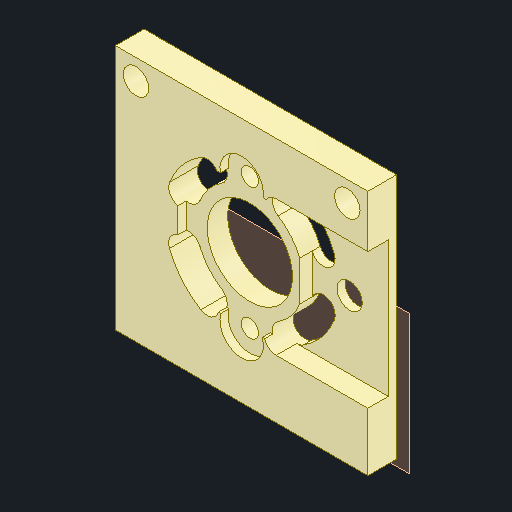
# Autodesk Inventor part: front_motur_holder
Saved by Autodesk Inventor 2023 (Build 270158000, 158)
## iProperties
Created: 2024-04-30
Part Number: front_motur_holder
Material: Nylon 6/6
Document SubType Name: Modeling
Designer: szymo
Density: 1.13 g/cm^3
Appearance: Nylon 6
Mass: 2.38963 g
Surface Area: 22.831 cm^2
Volume: 2.11472 cm^3
Author: szymo
Autodesk Inventor part; units mm, degrees
ref_plane "YZ Plane" through (0, 0, 0) normal (1, 0, 0) x (0, 1, 0)
ref_plane "XZ Plane" through (0, 0, 0) normal (0, 1, 0) x (-1, 0, 0)
ref_plane "XY Plane" through (0, 0, 0) normal (0, 0, 1) x (1, 0, 0)
ref_plane "Work Plane1" through (0, 0, 0) normal (0, 0, 1) x (1, 0, 0)
sketch "Sketch1" plane through (0, 0, 0) normal (0, 0, 1) x (1, 0, 0)
  arc A0 (-3.651, 13.5937) -> (-4.7619, 15.391) centre (-4.2064, 14.4923) ccw projected
  arc A1 (-3.651, 13.5937) -> (-6.4477, 10.2643) centre (0, 7.6875) ccw projected
  arc A2 (-8.4097, 11.0483) -> (-6.4477, 10.2643) centre (-7.4287, 10.6563) ccw projected
  arc A3 (-4.7619, 15.391) -> (-8.4097, 11.0483) centre (0, 7.6875) ccw projected
  arc A4 (6.4477, 10.2643) -> (8.4097, 11.0483) centre (7.4287, 10.6563) ccw projected
  arc A5 (6.4477, 10.2643) -> (3.651, 13.5937) centre (0, 7.6875) ccw projected
  arc A6 (4.7619, 15.391) -> (3.651, 13.5937) centre (4.2064, 14.4923) ccw projected
  arc A7 (8.4097, 11.0483) -> (4.7619, 15.391) centre (0, 7.6875) ccw projected
  arc A8 (-6.4563, 5.1322) -> (-8.4209, 4.3547) centre (-7.4386, 4.7434) ccw projected
  arc A9 (-6.4563, 5.1322) -> (-3.651, 1.7813) centre (0, 7.6875) ccw projected
  arc A10 (-4.7619, -0.016) -> (-3.651, 1.7813) centre (-4.2064, 0.8827) ccw projected
  arc A11 (-8.4209, 4.3547) -> (-4.7619, -0.016) centre (0, 7.6875) ccw projected
  arc A12 (3.651, 1.7813) -> (4.7619, -0.016) centre (4.2064, 0.8827) ccw projected
  arc A13 (3.651, 1.7813) -> (6.4563, 5.1322) centre (0, 7.6875) ccw projected
  arc A14 (8.4209, 4.3547) -> (6.4563, 5.1322) centre (7.4386, 4.7434) ccw projected
  arc A15 (4.7619, -0.016) -> (8.4209, 4.3547) centre (0, 7.6875) ccw projected
  circle A16 centre (10.65, 7.6999) radius 1.15 projected
  circle A17 centre (0, 15.6875) radius 1.0564 projected
  circle A18 centre (0, -0.3125) radius 1.0564 projected
  circle A19 centre (0, 7.6875) radius 5 projected
  circle A20 centre (0, 7.6875) radius 13.7 projected
  line L0 (-116.625, -11.1875) -> (15.375, -11.1875) projected
  line L1 (15.375, -11.1875) -> (15.375, -7.6875) projected
  line L2 (-116.625, -7.6875) -> (15.375, -7.6875) projected
  line L3 (-116.625, -11.1875) -> (-116.625, -7.6875) projected
  line L4 (15.375, -7.6875) -> (-15.375, -7.6875)
  line L5 (-15.375, -7.6875) -> (-15.375, 22.3125)
  line L6 (-15.375, 22.3125) -> (15.375, 22.3125)
  line L7 (15.375, 22.3125) -> (15.375, -7.6875)
  circle A21 centre (0, 7.6875) radius 14.375 projected
  circle A22 centre (0, 7.6875) radius 5.2
  arc A23 (-3.4406, 13.2535) -> (-4.9722, 15.7312) centre (-4.2064, 14.4923) ccw
  arc A24 (-3.4406, 13.2535) -> (-6.0763, 10.1158) centre (0, 7.6875) ccw
  arc A25 (-8.7812, 11.1968) -> (-6.0763, 10.1158) centre (-7.4287, 10.6563) ccw
  arc A26 (-4.9722, 15.7312) -> (-8.7812, 11.1968) centre (0, 7.6875) ccw
  arc A27 (4.9722, 15.7312) -> (3.4406, 13.2535) centre (4.2064, 14.4923) ccw
  arc A28 (6.0763, 10.1158) -> (3.4406, 13.2535) centre (0, 7.6875) ccw
  arc A29 (6.0763, 10.1158) -> (8.7812, 11.1968) centre (7.4287, 10.6563) ccw
  arc A30 (8.7812, 11.1968) -> (4.9722, 15.7312) centre (0, 7.6875) ccw
  arc A31 (3.4406, 2.1215) -> (6.0844, 5.2794) centre (0, 7.6875) ccw
  arc A32 (3.4406, 2.1215) -> (4.9722, -0.3562) centre (4.2064, 0.8827) ccw
  arc A33 (4.9722, -0.3562) -> (8.7928, 4.2075) centre (0, 7.6875) ccw
  arc A34 (8.7928, 4.2075) -> (6.0844, 5.2794) centre (7.4386, 4.7434) ccw
  arc A35 (-6.0844, 5.2794) -> (-8.7928, 4.2075) centre (-7.4386, 4.7434) ccw
  arc A36 (-6.0844, 5.2794) -> (-3.4406, 2.1215) centre (0, 7.6875) ccw
  arc A37 (-4.9722, -0.3562) -> (-3.4406, 2.1215) centre (-4.2064, 0.8827) ccw
  arc A38 (-8.7928, 4.2075) -> (-4.9722, -0.3562) centre (0, 7.6875) ccw
  circle A39 centre (10.65, 7.6999) radius 1.55
  point P0 (0, 0)
  dimension "d0" = 30
  dimension "d1" = 15.375
  dimension "d2" = 15.375
  dimension "d3" = 0.2
  dimension "d4" = 0.4
  dimension "d5" = 0.4
  dimension "d6" = 0.4
  dimension "d7" = 0.4
  dimension "d8" = 0.4
  constraints: 32 point on circle, 18 centre point, 8 end point, 2 parallel, 1 horizontal, 1 perpendicular, 12 other
  measures "d0" distance of L4.end L5.end
  measures "d1" distance from line of A3.centre L7
  measures "d2" distance from line of L5 A1.centre
  measures "d3" radial gap between concentric circles of A19 A22
  measures "d4" radial gap between concentric circles of A0 A23
  measures "d5" radial gap between concentric circles of A7 A30
  measures "d6" radial gap between concentric circles of A14 A34
  measures "d7" radial gap between concentric circles of A8 A35
  measures "d8" radial gap between concentric circles of A16 A39
extrude "Extrusion1" add sketch "Sketch1" along normal blind 1 contours A20 | L2 L5 L6 L7 | A21
sketch "Sketch2" plane through (0, 0, 1) normal (0, 0, 1) x (1, 0, 0)
  line L0 (15.375, 22.3125) -> (-15.375, 22.3125) projected
  line L1 (-15.375, 22.3125) -> (-15.375, -7.6875) projected
  line L2 (-15.375, -7.6875) -> (15.375, -7.6875) projected
  line L3 (15.375, -7.6875) -> (15.375, 22.3125) projected
  circle A0 centre (0, 15.6875) radius 1.0564 projected
  circle A1 centre (0, -0.3125) radius 1.0564 projected
  circle A2 centre (0, 7.6875) radius 5.2 projected
  arc A3 (-3.4406, 13.2535) -> (-6.0763, 10.1158) centre (0, 7.6875) ccw projected
  arc A4 (-8.7812, 11.1968) -> (-6.0763, 10.1158) centre (-7.4287, 10.6563) ccw projected
  arc A5 (-4.9722, 15.7312) -> (-8.7812, 11.1968) centre (0, 7.6875) ccw projected
  arc A6 (-3.4406, 13.2535) -> (-4.9722, 15.7312) centre (-4.2064, 14.4923) ccw projected
  arc A7 (6.0763, 10.1158) -> (3.4406, 13.2535) centre (0, 7.6875) ccw projected
  arc A8 (4.9722, 15.7312) -> (3.4406, 13.2535) centre (4.2064, 14.4923) ccw projected
  arc A9 (8.7812, 11.1968) -> (4.9722, 15.7312) centre (0, 7.6875) ccw projected
  arc A10 (6.0763, 10.1158) -> (8.7812, 11.1968) centre (7.4287, 10.6563) ccw projected
  arc A11 (3.4406, 2.1215) -> (4.9722, -0.3562) centre (4.2064, 0.8827) ccw projected
  arc A12 (3.4406, 2.1215) -> (6.0844, 5.2794) centre (0, 7.6875) ccw projected
  arc A13 (8.7928, 4.2075) -> (6.0844, 5.2794) centre (7.4386, 4.7434) ccw projected
  arc A14 (4.9722, -0.3562) -> (8.7928, 4.2075) centre (0, 7.6875) ccw projected
  arc A15 (-6.0844, 5.2794) -> (-3.4406, 2.1215) centre (0, 7.6875) ccw projected
  arc A16 (-4.9722, -0.3562) -> (-3.4406, 2.1215) centre (-4.2064, 0.8827) ccw projected
  arc A17 (-8.7928, 4.2075) -> (-4.9722, -0.3562) centre (0, 7.6875) ccw projected
  arc A18 (-6.0844, 5.2794) -> (-8.7928, 4.2075) centre (-7.4386, 4.7434) ccw projected
  circle A19 centre (10.65, 7.6999) radius 1.55 projected
  arc A20 (4.9722, 15.7312) -> (3.4406, 13.2535) centre (4.2064, 14.4923) ccw projected
  line L4 (4.2064, 15.9488) -> (15.375, 15.9488)
  line L5 (15.375, -7.6875) -> (15.375, 22.3125) projected
  line L6 (4.2064, -0.5738) -> (15.375, -0.5738)
  arc A21 (6.0763, 10.1158) -> (8.7812, 11.1968) centre (7.4287, 10.6563) ccw projected
  line L7 (6.0763, 10.1158) -> (6.0844, 5.2794)
  point P0 (0, 0)
  constraints: 6 end point, 2 perpendicular, 2 point on circle, 2 point on line, 1 tangent
extrude "Extrusion2" add sketch "Sketch2" along normal blind 1.5 contours L3 L4 A8 A7 L7 A12 A11 L6 L2 L1 L0
sketch "Sketch3" plane through (0, 0, 2.5) normal (0, 0, 1) x (1, 0, 0)
  line L0 (15.375, -7.6875) -> (15.375, -0.5738) projected
  line L1 (15.375, -0.5738) -> (4.2064, -0.5738) projected
  arc A0 (3.4406, 2.1215) -> (4.2064, -0.5738) centre (4.2064, 0.8827) ccw projected
  arc A1 (3.4406, 2.1215) -> (6.0844, 5.2794) centre (0, 7.6875) ccw projected
  line L2 (6.0844, 5.2794) -> (6.0763, 10.1158) projected
  arc A2 (6.0763, 10.1158) -> (3.4406, 13.2535) centre (0, 7.6875) ccw projected
  arc A3 (4.2064, 15.9488) -> (3.4406, 13.2535) centre (4.2064, 14.4923) ccw projected
  line L3 (4.2064, 15.9488) -> (15.375, 15.9488) projected
  line L4 (15.375, 15.9488) -> (15.375, 22.3125) projected
  line L5 (15.375, 22.3125) -> (-15.375, 22.3125) projected
  line L6 (-15.375, 22.3125) -> (-15.375, -7.6875) projected
  line L7 (-15.375, -7.6875) -> (15.375, -7.6875) projected
  circle A4 centre (0, 15.6875) radius 1.0564 projected
  circle A5 centre (0, -0.3125) radius 1.0564 projected
  arc A6 (-6.0844, 5.2794) -> (-8.7928, 4.2075) centre (-7.4386, 4.7434) ccw projected
  arc A7 (-6.0844, 5.2794) -> (-3.4406, 2.1215) centre (0, 7.6875) ccw projected
  arc A8 (-4.9722, -0.3562) -> (-3.4406, 2.1215) centre (-4.2064, 0.8827) ccw projected
  arc A9 (-8.7928, 4.2075) -> (-4.9722, -0.3562) centre (0, 7.6875) ccw projected
  arc A10 (-3.4406, 13.2535) -> (-4.9722, 15.7312) centre (-4.2064, 14.4923) ccw projected
  arc A11 (-3.4406, 13.2535) -> (-6.0763, 10.1158) centre (0, 7.6875) ccw projected
  arc A12 (-8.7812, 11.1968) -> (-6.0763, 10.1158) centre (-7.4287, 10.6563) ccw projected
  arc A13 (-4.9722, 15.7312) -> (-8.7812, 11.1968) centre (0, 7.6875) ccw projected
  circle A14 centre (0, 7.6875) radius 5.2 projected
  circle A15 centre (0, 15.6875) radius 2.65
  circle A16 centre (0, -0.3125) radius 1.0564 projected
  circle A17 centre (0, -0.3125) radius 2.65
  arc A18 (-2.4425, 10.6818) -> (-4.3563, 11.5819) centre (-5.3868, 6.906) ccw projected
  arc A19 (-4.3563, 11.5819) -> (-4.9119, 10.8525) centre (0, 7.6875) ccw projected
  arc A20 (-4.9119, 10.8525) -> (-3.5356, 9.2466) centre (-0.678, 13.0883) ccw projected
  arc A21 (-3.5356, 9.2466) -> (-3.736, 8.6743) centre (0, 7.6875) ccw projected
  arc A22 (-3.736, 8.6743) -> (-5.8134, 8.2775) centre (-3.8987, 3.889) ccw projected
  arc A23 (-5.8134, 8.2775) -> (-5.8341, 7.3609) centre (0, 7.6875) ccw projected
  arc A24 (-5.8341, 7.3609) -> (-3.7768, 6.8706) centre (-3.723, 11.6584) ccw projected
  arc A25 (-3.7768, 6.8706) -> (-3.6025, 6.2899) centre (0, 7.6875) ccw projected
  arc A26 (-3.6025, 6.2899) -> (-5.05, 4.7478) centre (-0.9214, 2.3228) ccw projected
  arc A27 (-5.05, 4.7478) -> (-4.5279, 3.994) centre (0, 7.6875) ccw projected
  arc A28 (-4.5279, 3.994) -> (-2.5753, 4.8067) centre (-5.346, 8.7117) ccw projected
  arc A29 (-2.5753, 4.8067) -> (-2.093, 4.4393) centre (0, 7.6875) ccw projected
  arc A30 (-2.093, 4.4393) -> (-2.3576, 2.341) centre (2.4078, 2.8058) ccw projected
  arc A31 (-2.3576, 2.341) -> (-1.4922, 2.038) centre (0, 7.6875) ccw projected
  arc A32 (-1.4922, 2.038) -> (-0.3902, 3.8431) centre (-4.927, 5.3738) ccw projected
  arc A33 (-0.3902, 3.8431) -> (0.216, 3.8294) centre (0, 7.6875) ccw projected
  arc A34 (0.216, 3.8294) -> (1.2353, 1.9763) centre (4.8174, 5.1534) ccw projected
  arc A35 (1.2353, 1.9763) -> (2.1135, 2.2398) centre (0, 7.6875) ccw projected
  arc A36 (2.1135, 2.2398) -> (1.944, 4.348) centre (-2.6261, 2.9196) ccw projected
  arc A37 (1.944, 4.348) -> (2.4425, 4.6932) centre (0, 7.6875) ccw projected
  arc A38 (2.4425, 4.6932) -> (4.3563, 3.7931) centre (5.3868, 8.469) ccw projected
  arc A39 (4.3563, 3.7931) -> (4.9119, 4.5225) centre (0, 7.6875) ccw projected
  arc A40 (4.9119, 4.5225) -> (3.5356, 6.1284) centre (0.678, 2.2867) ccw projected
  arc A41 (3.5356, 6.1284) -> (3.736, 6.7007) centre (0, 7.6875) ccw projected
  arc A42 (3.736, 6.7007) -> (5.8134, 7.0975) centre (3.8987, 11.486) ccw projected
  arc A43 (5.8134, 7.0975) -> (5.8341, 8.0141) centre (0, 7.6875) ccw projected
  arc A44 (5.8341, 8.0141) -> (3.7768, 8.5044) centre (3.723, 3.7166) ccw projected
  arc A45 (3.7768, 8.5044) -> (3.6025, 9.0851) centre (0, 7.6875) ccw projected
  arc A46 (3.6025, 9.0851) -> (5.05, 10.6272) centre (0.9214, 13.0522) ccw projected
  arc A47 (5.05, 10.6272) -> (4.5279, 11.381) centre (0, 7.6875) ccw projected
  arc A48 (4.5279, 11.381) -> (2.5753, 10.5683) centre (5.346, 6.6633) ccw projected
  arc A49 (2.5753, 10.5683) -> (2.093, 10.9357) centre (0, 7.6875) ccw projected
  arc A50 (2.093, 10.9357) -> (2.3576, 13.034) centre (-2.4078, 12.5692) ccw projected
  arc A51 (2.3576, 13.034) -> (1.4922, 13.337) centre (0, 7.6875) ccw projected
  arc A52 (1.4922, 13.337) -> (0.3902, 11.5319) centre (4.927, 10.0012) ccw projected
  arc A53 (0.3902, 11.5319) -> (-0.216, 11.5456) centre (0, 7.6875) ccw projected
  arc A54 (-0.216, 11.5456) -> (-1.2353, 13.3987) centre (-4.8174, 10.2216) ccw projected
  arc A55 (-1.2353, 13.3987) -> (-2.1135, 13.1352) centre (0, 7.6875) ccw projected
  arc A56 (-2.1135, 13.1352) -> (-1.944, 11.027) centre (2.6261, 12.4554) ccw projected
  arc A57 (-1.944, 11.027) -> (-2.4425, 10.6818) centre (0, 7.6875) ccw projected
  circle A58 centre (0, 7.6875) radius 5.8433
  circle A59 centre (0, 7.6875) radius 6.5436
  arc A60 (-3.4406, 13.2535) -> (-4.9722, 15.7312) centre (-4.2064, 14.4923) ccw projected
  line L8 (-2.9676, 15.2581) -> (-2.615, 15.2581)
  arc A61 (4.9722, 15.7312) -> (3.4406, 13.2535) centre (4.2064, 14.4923) ccw projected
  line L9 (2.9676, 15.2581) -> (2.615, 15.2581)
  arc A62 (3.4406, 2.1215) -> (4.9722, -0.3562) centre (4.2064, 0.8827) ccw projected
  line L10 (2.8055, 0.4846) -> (2.5273, 0.4846)
  arc A63 (-4.9722, -0.3562) -> (-3.4406, 2.1215) centre (-4.2064, 0.8827) ccw projected
  line L11 (-2.8055, 0.4846) -> (-2.5273, 0.4846)
  arc A64 (-8.7812, 11.1968) -> (-6.0763, 10.1158) centre (-7.4287, 10.6563) ccw projected
  line L12 (-7.7556, 9.237) -> (-7.7556, 6.165)
  point P0 (0, 0)
  point P1 (-6.0844, 5.2794)
  point P2 (-6.0763, 10.1158)
  point P3 (2.9676, 15.2581)
  dimension "d13" = 5.3
  dimension "d14" = 5.3
  constraints: 12 point on circle, 10 end point, 4 centre point, 4 coincident, 4 point on line, 1 concentric, 1 horizontal, 1 parallel, 1 vertical
  measures "d13" diameter of A15
  measures "d14" diameter of A17
extrude "Extrusion3" add sketch "Sketch3" along normal blind 1 contours L7 L6 L5 L4 L3 A3 L9 A15 L8 A10 A13 A12 L12 A6 A9 A8 L11 A17 L10 A0 L1 L0
sketch "Sketch5" plane through (0, 0, 0) normal (0, 0, -1) x (-1, 0, 0)
  line L0 (-15.375, 22.3125) -> (15.375, 22.3125) projected
  line L1 (-15.375, -7.6875) -> (-15.375, 22.3125) projected
  line L2 (15.375, -7.6875) -> (-15.375, -7.6875) projected
  line L3 (15.375, 22.3125) -> (15.375, -7.6875) projected
  circle A0 centre (0, 15.6875) radius 1.0564 projected
  circle A1 centre (0, -0.3125) radius 1.0564 projected
  circle A2 centre (0, 7.6875) radius 5.2 projected
  arc A3 (6.0763, 10.1158) -> (3.4406, 13.2535) centre (0, 7.6875) ccw projected
  arc A4 (4.9722, 15.7312) -> (3.4406, 13.2535) centre (4.2064, 14.4923) ccw projected
  arc A5 (8.7812, 11.1968) -> (4.9722, 15.7312) centre (0, 7.6875) ccw projected
  arc A6 (6.0763, 10.1158) -> (8.7812, 11.1968) centre (7.4287, 10.6563) ccw projected
  arc A7 (-3.4406, 13.2535) -> (-6.0763, 10.1158) centre (0, 7.6875) ccw projected
  arc A8 (-8.7812, 11.1968) -> (-6.0763, 10.1158) centre (-7.4287, 10.6563) ccw projected
  arc A9 (-4.9722, 15.7312) -> (-8.7812, 11.1968) centre (0, 7.6875) ccw projected
  arc A10 (-3.4406, 13.2535) -> (-4.9722, 15.7312) centre (-4.2064, 14.4923) ccw projected
  arc A11 (-4.9722, -0.3562) -> (-3.4406, 2.1215) centre (-4.2064, 0.8827) ccw projected
  arc A12 (-8.7928, 4.2075) -> (-4.9722, -0.3562) centre (0, 7.6875) ccw projected
  arc A13 (-6.0844, 5.2794) -> (-8.7928, 4.2075) centre (-7.4386, 4.7434) ccw projected
  arc A14 (-6.0844, 5.2794) -> (-3.4406, 2.1215) centre (0, 7.6875) ccw projected
  arc A15 (3.4406, 2.1215) -> (6.0844, 5.2794) centre (0, 7.6875) ccw projected
  arc A16 (8.7928, 4.2075) -> (6.0844, 5.2794) centre (7.4386, 4.7434) ccw projected
  arc A17 (4.9722, -0.3562) -> (8.7928, 4.2075) centre (0, 7.6875) ccw projected
  arc A18 (3.4406, 2.1215) -> (4.9722, -0.3562) centre (4.2064, 0.8827) ccw projected
  circle A19 centre (-10.65, 7.6999) radius 1.55 projected
  circle A20 centre (-12.875, 19.8125) radius 2.5
  circle A21 centre (12.875, 19.8125) radius 2.5
  point P0 (0, 0)
  dimension "d26" = 5
  dimension "d27" = 5
  dimension "d28" = 2.5
  dimension "d29" = 2.5
  dimension "d30" = 2.5
  dimension "d31" = 2.5
  constraints: 2 centre point, 2 coincident
  measures "d26" diameter of A20
  measures "d27" diameter of A21
  measures "d28" distance from line of L0 A20.centre
  measures "d29" distance from line of L1 A20.centre
  measures "d30" distance from line of L0 A21.centre
  measures "d31" distance from line of L3 A21.centre
hole "Hole2" at (12.875, 19.8125, 0) at (-12.875, 19.8125, 0) direction (0, 0, 1) diameter 3.1 end through all countersink diameter 5 countersink angle 90 clearance for "Countersunk Flat Head Screw ISO 2009/7046" size "M2.5" standard "ISO"
equation "\"d2\" = d1"
equation "\"d28\" = 0.5 * d26"
equation "\"d29\" = 0.5 * d26"
equation "\"d30\" = 0.5 * d27"
equation "\"d31\" = 0.5 * d27"
body "Solid1"
